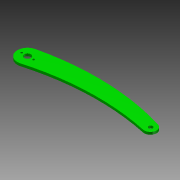
# Autodesk Inventor part: brazo
Saved by Autodesk Inventor 2012 (Build 160160000, 160)
## iProperties
Created: 2013-10-01
Part Number: brazo
Material: Default
Document SubType Name: Modeling
Designer: Nick
Density: 1 g/cm^3
Author: Nick
Autodesk Inventor part; units mm, degrees
ref_plane "YZ Plane" through (0, 0, 0) normal (1, 0, 0) x (0, 1, 0)
ref_plane "XZ Plane" through (0, 0, 0) normal (0, 1, 0) x (-1, 0, 0)
ref_plane "XY Plane" through (0, 0, 0) normal (0, 0, 1) x (1, 0, 0)
sketch "Sketch1" plane through (0, 0, 0) normal (0, 0, 1) x (1, 0, 0)
  line L0 (0, 0) -> (150, 0) construction
  circle A0 centre (0, 0) radius 4
  circle A1 centre (0, 0) radius 12.5 construction
  circle A2 centre (150, 0) radius 2.5
  circle A3 centre (150, 0) radius 7.5 construction
  arc A4 (150, 0) -> (0, 0) centre (75, -290.4738) ccw construction
  line L1 (-4.0971, 17.3539) -> (0, 0) construction
  line L2 (0, 0) -> (12.1656, 2.8722) construction
  line L3 (0, 0) -> (3.4621, -14.6644) construction
  line L4 (147.6861, -9.448) -> (150, 0) construction
  line L5 (150, 0) -> (152.7079, 11.057) construction
  line L6 (150, 0) -> (150, 0) construction
  line L7 (150, 0) -> (142.7153, 1.7841) construction
  arc A5 (151.7841, 7.2847) -> (-2.8722, 12.1656) centre (65.313, -279.983) ccw
  arc A6 (148.2159, -7.2847) -> (2.8722, -12.1656) centre (85.3125, -300.6159) ccw
  arc A7 (-2.8722, 12.1656) -> (2.8722, -12.1656) centre (-0.0311, -0.0073) ccw
  arc A8 (148.2159, -7.2847) -> (151.7841, 7.2847) centre (149.6194, 0.0932) ccw
  circle A9 centre (-0.0311, -0.0073) radius 7.25 construction
  circle A10 centre (-7.2811, 0) radius 1.25
  circle A11 centre (7.2189, 0) radius 1.25
  dimension "d0" = 150
  dimension "d1" = 8
  dimension "d2" = 25
  dimension "d3" = 5
  dimension "d4" = 15
  dimension "d6" = 300
  dimension "d7" = 90
  dimension "d8" = 180
  dimension "d9" = 180
  dimension "d10" = 90
  dimension "d11" = 300
  dimension "d12" = 300
  dimension "d13" = 14.5
  dimension "d14" = 2.5
  dimension "d15" = 2.5
  constraints: 21 point on circle, 16 end point, 12 centre point, 5 coincident, 5 point on line, 3 tangent, 1 horizontal, 1 horizontal alignment
  measures "d0" distance of L0.start L0.end
  measures "d1" diameter of A0
  measures "d2" diameter of A1
  measures "d3" diameter of A2
  measures "d4" diameter of A3
  measures "d6" radius of A4
  measures "d7" angle of L2 L1
  measures "d8" angle of L3 L1
  measures "d9" angle of L5 L4
  measures "d10" angle of L7 L5
  measures "d11" radius of A5
  measures "d12" radius of A6
  measures "d13" diameter of A9
  measures "d14" diameter of A10
  measures "d15" diameter of A11
extrude "Extrusion1" add sketch "Sketch1" along normal blind 3
body "Solid1"
